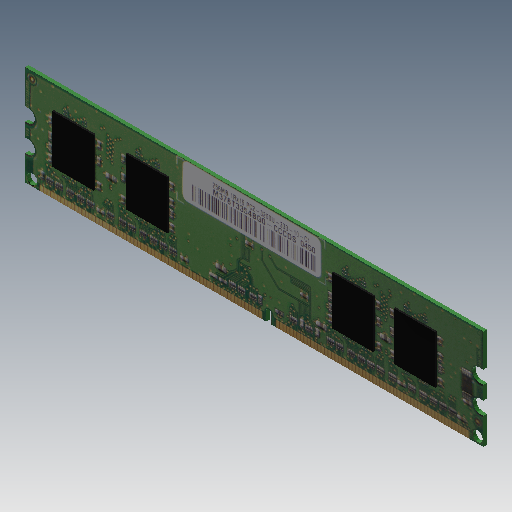
# Autodesk Inventor part: config - ram
Saved by Autodesk Inventor 2020 (Build 240152000, 152)
## iProperties
Created: 2005-12-12
Part Number: config - ram
Document SubType Name: Modeling
Designer: Simon.Ng@autodesk.com
Stock Number: config - ram
Density: 1 g/cm^3
Material: Generic
Mass: 4.45281 g
Surface Area: 81.6838 cm^2
Volume: 4.45281 cm^3
Appearance: Smooth - Dark Forest Green
Company: Autodesk Asia Pte. Ltd.
Title: PC Demo
Author: Simon.Ng@autodesk.com
Autodesk Inventor part; units mm, degrees
ref_plane "YZ Plane" through (0, 0, 0) normal (1, 0, 0) x (0, 1, 0)
ref_plane "XZ Plane" through (0, 0, 0) normal (0, 1, 0) x (-1, 0, 0)
ref_plane "XY Plane" through (0, 0, 0) normal (0, 0, 1) x (1, 0, 0)
sketch "Sketch1" plane through (0, 0, 0) normal (0, 0, 1) x (1, 0, 0)
  line L0 (0, 37.7) -> (0, -2.9) projected
  line L1 (-79.8, 0) -> (106.4, 0) projected
  line L2 (-66.5, 0) -> (66.5, 0)
  line L3 (66.5, 0) -> (66.5, 29)
  line L4 (66.5, 29) -> (-66.5, 29)
  line L5 (-66.5, 29) -> (-66.5, 0)
  dimension "d0" = 133
  dimension "d1" = 29
  constraints: 8 end point, 2 parallel, 1 horizontal, 1 perpendicular, 1 point on line, 1 other
  measures "d0" distance of L3.end L4.end
  measures "d1" distance of L4.end L2.start
extrude "Extrusion1" add sketch "Sketch1" along normal blind 1
decal "Decal1"
decal "Decal2"
sketch "Sketch5" plane through (0, 0, 1) normal (0, 0, 1) x (1, 0, 0)
  line L0 (-66.5, 0) -> (-66.5, 29) projected
  line L1 (66.5, 29) -> (66.5, 0) projected
  line L2 (-66.5, 19.147) -> (-65.5825, 19.147)
  line L3 (-65.5825, 19.147) -> (-65.5825, 15.2864)
  line L4 (-65.5825, 15.2864) -> (-66.5, 15.2864)
  line L5 (-66.5, 15.2864) -> (-66.5, 19.147)
  line L6 (-66.5, 11.2859) -> (-65.5825, 11.2859)
  line L7 (-65.5825, 11.2859) -> (-65.5825, 7.4252)
  line L8 (-65.5825, 7.4252) -> (-66.5, 7.4252)
  line L9 (-66.5, 7.4252) -> (-66.5, 11.2859)
  circle A0 centre (-65.5825, 17.2167) radius 1.9303
  circle A1 centre (-65.5825, 9.3555) radius 1.9303
  line L10 (66.5, 19.4238) -> (65.1393, 19.4238)
  line L11 (65.1393, 19.4238) -> (65.1393, 15.6247)
  line L12 (65.1393, 15.6247) -> (66.5, 15.6247)
  line L13 (66.5, 15.6247) -> (66.5, 19.4238)
  line L14 (66.5, 11.6256) -> (65.3393, 11.6256)
  line L15 (65.3393, 11.6256) -> (65.3393, 7.8264)
  line L16 (65.3393, 7.8264) -> (66.5, 7.8264)
  line L17 (66.5, 7.8264) -> (66.5, 11.6256)
  circle A2 centre (65.1393, 17.5243) radius 1.8996
  circle A3 centre (65.3393, 9.726) radius 1.8996
  circle A4 centre (-64.4646, 1.8448) radius 1.5
  circle A5 centre (64.8231, 1.8448) radius 1.5
  dimension "d12" = 3
  constraints: 32 end point, 8 parallel, 4 horizontal, 4 midpoint, 4 perpendicular, 4 point on line, 4 vertical alignment, 2 centre point, 1 equal radius, 1 horizontal alignment, 8 other
  measures "d12" diameter of A4
extrude "Extrusion2" cut sketch "Sketch5" against normal through all
sketch "Sketch6" plane through (0, 0, 1) normal (0, 0, 1) x (1, 0, 0)
  line L0 (66.5, 0) -> (-66.5, 0) projected
  line L1 (3.433, 2.75) -> (4.933, 2.75)
  line L2 (4.933, 2.75) -> (4.933, 0)
  line L3 (4.933, 0) -> (3.433, 0)
  line L4 (3.433, 0) -> (3.433, 2.75)
  circle A0 centre (4.183, 2.75) radius 0.75
  dimension "d15" = 1.5
  dimension "d16" = 2.75
  constraints: 8 end point, 2 parallel, 1 horizontal, 1 horizontal alignment, 1 midpoint, 1 perpendicular, 1 point on line, 2 other
  measures "d15" distance between parallel lines of L2 L4
  measures "d16" distance between parallel lines of L0 L1
extrude "Extrusion3" cut sketch "Sketch6" against normal through all
sketch "Sketch7" plane through (0, 0, 1) normal (0, 0, 1) x (1, 0, 0)
  line L0 (-46.1031, 8.3659) -> (-58.1031, 8.3659)
  line L1 (-58.1031, 8.3659) -> (-58.1031, 22.3659)
  line L2 (-58.1031, 22.3659) -> (-46.1031, 22.3659)
  line L3 (-46.1031, 22.3659) -> (-46.1031, 8.3659)
  line L4 (-36.7296, 22.3659) -> (-24.7296, 22.3659)
  line L5 (-24.7296, 22.3659) -> (-24.7296, 8.3659)
  line L6 (-24.7296, 8.3659) -> (-36.7296, 8.3659)
  line L7 (-36.7296, 8.3659) -> (-36.7296, 22.3659)
  line L8 (22.9991, 22.3659) -> (34.9991, 22.3659)
  line L9 (34.9991, 22.3659) -> (34.9991, 8.3659)
  line L10 (34.9991, 8.3659) -> (22.9991, 8.3659)
  line L11 (22.9991, 8.3659) -> (22.9991, 22.3659)
  line L12 (40.9859, 22.3659) -> (52.9859, 22.3659)
  line L13 (52.9859, 22.3659) -> (52.9859, 8.3659)
  line L14 (52.9859, 8.3659) -> (40.9859, 8.3659)
  line L15 (40.9859, 8.3659) -> (40.9859, 22.3659)
  dimension "d21" = 14
  dimension "d22" = 12
  constraints: 32 end point, 9 collinear, 8 parallel, 4 horizontal, 4 perpendicular
  measures "d21" distance of L0.end L1.end
  measures "d22" distance of L1.end L2.end
extrude "Extrusion4" add sketch "Sketch7" along normal blind 0.5
sketch "Sketch8" plane through (0, 0, 0) normal (0, 0, -1) x (-1, 0, 0)
  line L0 (-58.0858, 22.4822) -> (-46.5858, 22.4822)
  line L1 (-46.5858, 22.4822) -> (-46.5858, 8.4822)
  line L2 (-46.5858, 8.4822) -> (-58.0858, 8.4822)
  line L3 (-58.0858, 8.4822) -> (-58.0858, 22.4822)
  line L4 (-36.8395, 22.4822) -> (-25.3395, 22.4822)
  line L5 (-25.3395, 22.4822) -> (-25.3395, 8.4822)
  line L6 (-25.3395, 8.4822) -> (-36.8395, 8.4822)
  line L7 (-36.8395, 8.4822) -> (-36.8395, 22.4822)
  line L8 (23.4032, 22.2455) -> (34.9032, 22.2455)
  line L9 (34.9032, 22.2455) -> (34.9032, 8.4822)
  line L10 (34.9032, 8.4822) -> (23.4032, 8.4822)
  line L11 (23.4032, 8.4822) -> (23.4032, 22.2455)
  line L12 (41.476, 22.1379) -> (52.976, 22.1379)
  line L13 (52.976, 22.1379) -> (52.976, 8.4822)
  line L14 (52.976, 8.4822) -> (41.476, 8.4822)
  line L15 (41.476, 8.4822) -> (41.476, 22.1379)
  dimension "d28" = 11.5
  dimension "d29" = 14
  constraints: 32 end point, 8 parallel, 4 collinear, 4 horizontal, 4 perpendicular, 3 equal length
  measures "d28" distance of L0.start L0.end
  measures "d29" distance of L2.end L0.start
extrude "Extrusion5" add sketch "Sketch8" along normal blind 0.5
sketch "Sketch3" plane through (0, 0, 1) normal (0, 0, 1) x (1, 0, 0)
  line L0 (-66.5, 29) -> (66.5, 29) construction
  line L1 (66.5, 29) -> (66.5, -0.391) construction
  line L2 (66.5, -0.391) -> (-66.5, -0.391) construction
  line L3 (-66.5, -0.391) -> (-66.5, 29) construction
  constraints: 2 other
sketch "Sketch4" plane through (0, 0, 0) normal (0, 0, -1) x (-1, 0, 0)
  line L0 (-66.5, 29) -> (66.5, 29) construction
  line L1 (66.5, 29) -> (66.5, -0.391) construction
  line L2 (66.5, -0.391) -> (-66.5, -0.391) construction
  line L3 (-66.5, -0.391) -> (-66.5, 29) construction
  constraints: 2 other
body "Solid1"
